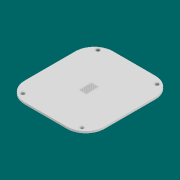
# Autodesk Inventor part: pcb
Saved by Autodesk Inventor 2020 (Build 240168000, 168)
## iProperties
Created: 2025-05-06
Part Number: pcb
Material: Generico
Document SubType Name: Modeling
Designer: Nicola Milia
Density: 1 g/cm^3
Appearance: Default
Author: Nicola Milia
Autodesk Inventor part; units mm, degrees
ref_plane "YZ Plane" through (0, 0, 0) normal (1, 0, 0) x (0, 1, 0)
ref_plane "XZ Plane" through (0, 0, 0) normal (0, 1, 0) x (-1, 0, 0)
ref_plane "XY Plane" through (0, 0, 0) normal (0, 0, 1) x (1, 0, 0)
sketch "Schizzo1" plane through (0, 0, 0) normal (0, 1, 0) x (-1, 0, 0)
  line L0 (20, 0) -> (65, 0)
  line L1 (85, -20) -> (85, -74)
  line L2 (65, -94) -> (20, -94)
  line L3 (0, -74) -> (0, -20)
  arc A0 (85, -20) -> (65, 0) centre (65, -20) ccw
  arc A1 (20, 0) -> (0, -20) centre (20, -20) ccw
  arc A2 (0, -74) -> (20, -94) centre (20, -74) ccw
  arc A3 (65, -94) -> (85, -74) centre (65, -74) ccw
  circle A4 centre (74, -7) radius 1.75
  circle A5 centre (74, -87) radius 1.75
  circle A6 centre (11, -87) radius 1.75
  circle A7 centre (11, -7) radius 1.75
  circle A8 centre (46.5, -41.3) radius 0.5
  circle A9 centre (46.5, -43.2) radius 0.5
  circle A10 centre (46.5, -45.1) radius 0.5
  circle A11 centre (46.5, -47) radius 0.5
  circle A12 centre (46.5, -48.9) radius 0.5
  circle A13 centre (46.5, -50.8) radius 0.5
  circle A14 centre (46.5, -52.7) radius 0.5
  circle A15 centre (44.6, -41.3) radius 0.5
  circle A16 centre (44.6, -43.2) radius 0.5
  circle A17 centre (44.6, -45.1) radius 0.5
  circle A18 centre (44.6, -47) radius 0.5
  circle A19 centre (44.6, -48.9) radius 0.5
  circle A20 centre (44.6, -50.8) radius 0.5
  circle A21 centre (44.6, -52.7) radius 0.5
  circle A22 centre (42.7, -41.3) radius 0.5
  circle A23 centre (42.7, -43.2) radius 0.5
  circle A24 centre (42.7, -45.1) radius 0.5
  circle A25 centre (42.7, -47) radius 0.5
  circle A26 centre (42.7, -48.9) radius 0.5
  circle A27 centre (42.7, -50.8) radius 0.5
  circle A28 centre (42.7, -52.7) radius 0.5
  circle A29 centre (40.8, -41.3) radius 0.5
  circle A30 centre (40.8, -43.2) radius 0.5
  circle A31 centre (40.8, -45.1) radius 0.5
  circle A32 centre (40.8, -47) radius 0.5
  circle A33 centre (40.8, -48.9) radius 0.5
  circle A34 centre (40.8, -50.8) radius 0.5
  circle A35 centre (40.8, -52.7) radius 0.5
  point P0 (46.5, -48.9)
  point P1 (46.5, -48.9)
  point P2 (44.6, -48.9)
  point P3 (42.7, -48.9)
  point P4 (40.8, -48.9)
  dimension "d20" = 3.5
  dimension "d21" = 3.5
  dimension "d22" = 3.5
  dimension "d23" = 3.5
  dimension "d29" = 1.9
  dimension "d32" = 1.9
  dimension "d37" = 1.9
  dimension "d40" = 1.9
  dimension "d43" = 1
  dimension "d46" = 1.9
  dimension "d49" = 1.9
  constraints: 36 centre point, 8 end point, 8 point on circle, 8 tangent, 4 horizontal, 3 equal radius, 3 vertical, 2 parallel, 1 coincident, 1 perpendicular, 84 other
  measures "d20" diameter of A4
  measures "d21" diameter of A5
  measures "d22" diameter of A6
  measures "d23" diameter of A7
  measures "d29" distance of point (46.5, -47) point (46.5, -48.9)
  measures "d32" distance of point (46.5, -47) point (44.6, -47)
  measures "d37" distance of point (46.5, -47) point (46.5, -45.1)
  measures "d40" distance of point (46.5, -47) point (44.6, -47)
  measures "d43" diameter of A8
  measures "d46" distance of A8.centre A9.centre
  measures "d49" distance of A8.centre A15.centre
extrude "Estrusione1" add sketch "Schizzo1" along normal blind 1.8
